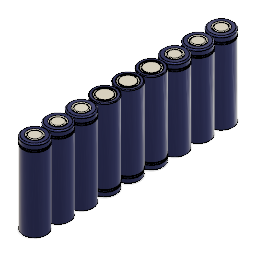
18650 Li-ion Battery Pack (Autodesk Fusion 360 design; units mm, degrees)
description: 3.2V 3000 mAh
description: 3000 mAh
part number: Samsung 30Q
Autodesk Fusion 360 part; units mm, degrees
sketch "Sketch1" plane through (0, 0, 0) normal (0, 1, 0) x (1, 0, 0)
  circle A0 centre (0, 0) radius 9.3
  dimension "d1" = 18.6
  constraint coincident A0.centre origin
  measures "d1" diameter of A0
extrude "Extrude1" add sketch "Sketch1" along normal blind 65.3 makes body 1
sketch "Sketch2" plane through (0, 0, 0) normal (0, -1, 0) x (1, 0, 0)
  circle A0 centre (0, 0) radius 9.3
torus "TorusPrimitive2" cut centre line diameter 12.5 section diameter 1 placed x (1, 0, 0) y (0, 0, 1) z (0, -1, 0) at (0, 0, 0) bodies 1
fillet "Fillet1" radius 0.5 3 edges at (-8.6706, 0, 3.363) (2.4409, 0, 6.2932) (-2.0793, 0, 5.3609) on bodies 1
torus "TorusPrimitive3" add centre line diameter 18.6 section diameter 1 placed x (-1, 0, 0) y (0, 0, 1) z (0, 1, 0) at (0, 65.3, 0) separate body makes body 2
move_body "MoveFace1" bodies 2 to x (1, 0, 0) y (0, 1, 0) z (0, 0, 1) at (0, -5, 0) on bodies 2
combine "Combine1" operation cut target body 1 tool bodies 2
fillet "Fillet4" radius 0.5 2 edges at (-8.6706, 59.8, -3.363) (-8.6706, 60.8, 3.363) on bodies 1
fillet "Fillet5" radius 1 1 edges at (-8.6706, 65.3, 3.363) on bodies 1
torus "TorusPrimitive4" cut centre line diameter 10.5 section diameter 1 placed x (-1, 0, 0) y (0, 0, 1) z (0, 1, 0) at (0, 65.3, 0) bodies 1
fillet "Fillet7" radius 1 1 edges at (-1.7177, 65.3, -4.4286) on bodies 1
copy_body "Body->Comp1" bodies 1 removing the originals makes body 3 in component "Battery"
pattern_linear "5" [suppressed]
component "Battery" placed x (1, 0, 0) y (0, 1, 0) z (0, 0, 1) at (0, 0, 0)
component "Battery" placed x (1, 0, 0) y (0, 1, 0) z (0, 0, 1) at (0, 0, -74.4)
component "Battery" placed x (1, 0, 0) y (0, 1, 0) z (0, 0, 1) at (0, 0, -55.8)
component "Battery" placed x (1, 0, 0) y (0, 1, 0) z (0, 0, 1) at (0, 0, -37.2)
component "Battery" placed x (1, 0, 0) y (0, 1, 0) z (0, 0, 1) at (0, 0, -18.6)
component "Battery" placed x (1, 0, 0) y (0, 1, 0) z (0, 0, 1) at (0, 0, 18.6)
component "Battery" placed x (1, 0, 0) y (0, 1, 0) z (0, 0, 1) at (0, 0, 37.2)
component "Battery" placed x (1, 0, 0) y (0, 1, 0) z (0, 0, 1) at (0, 0, 55.8)
component "Battery" placed x (1, 0, 0) y (0, 1, 0) z (0, 0, 1) at (0, 0, 74.4)
